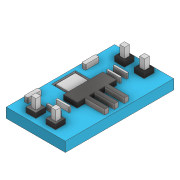
# Autodesk Inventor part: ghj
Saved by Autodesk Inventor 2021 (Build 250183000, 183)
## iProperties
Created: 2021-07-12
Part Number: ghj
Material: Generic
Document SubType Name: Modeling
Designer: Shaheen Khan
Density: 1 g/cm^3
Appearance: Default
Author: Shaheen Khan
Autodesk Inventor part; units mm, degrees
ref_plane "YZ Plane" through (0, 0, 0) normal (1, 0, 0) x (0, 1, 0)
ref_plane "XZ Plane" through (0, 0, 0) normal (0, 1, 0) x (-1, 0, 0)
ref_plane "XY Plane" through (0, 0, 0) normal (0, 0, 1) x (1, 0, 0)
sketch "Sketch1" plane through (0, 0, 0) normal (0, 1, 0) x (-1, 0, 0)
  line L0 (-15, 27.5) -> (15, 27.5)
  line L1 (15, 27.5) -> (15, -27.5)
  line L2 (15, -27.5) -> (-15, -27.5)
  line L3 (-15, -27.5) -> (-15, 27.5)
  line L4 (-15, 27.5) -> (15, -27.5) construction
  line L5 (15, 27.5) -> (-15, -27.5) construction
  point P0 (0, 0)
  dimension "d0" = 55
  dimension "d1" = 30
  constraints: 12 end point, 2 midpoint, 2 parallel, 1 horizontal, 1 perpendicular
  measures "d0" distance of L0.end L1.end
  measures "d1" distance of L1.end L2.end
extrude "Extrusion1" add sketch "Sketch1" along normal blind 5
sketch "Sketch2" plane through (0, 5, 0) normal (0, 1, 0) x (1, 0, 0)
  line L0 (-7.5, -25) -> (-2.5, -25)
  line L1 (-2.5, -25) -> (-2.5, -20)
  line L2 (-2.5, -20) -> (-7.5, -20)
  line L3 (-7.5, -20) -> (-7.5, -25)
  line L4 (-7.5, -25) -> (-2.5, -20) construction
  line L5 (-2.5, -25) -> (-7.5, -20) construction
  line L6 (-21.5261, -24.4969) -> (-16.5342, -20) construction
  line L7 (-15.0081, -24.7484) -> (-20, -20.2516) construction
  line L8 (-4.2253, 22.2548) -> (-1.8361, 26.5023) construction
  line L9 (-1.8361, 22.2548) -> (-4.2253, 26.5023) construction
  line L10 (-16.2912, 21.4805) -> (-13.725, 24.9537) construction
  line L11 (-13.725, 21.4805) -> (-16.2912, 24.9537) construction
  line L12 (-15, -27.5) -> (15, -27.5) projected
  line L13 (2.5, -25) -> (7.5, -25)
  line L14 (7.5, -25) -> (7.5, -20)
  line L15 (7.5, -20) -> (2.5, -20)
  line L16 (2.5, -20) -> (2.5, -25)
  line L17 (2.5, -25) -> (7.5, -20) construction
  line L18 (7.5, -25) -> (2.5, -20) construction
  point P0 (0, 0)
  point P1 (-5, -22.5)
  point P2 (-3.0307, 24.3785)
  point P3 (5, -22.5)
  dimension "d4" = 5
  dimension "d7" = 5
  dimension "d8" = 5
  dimension "d9" = 5
  dimension "d10" = 5
  dimension "d11" = 5
  dimension "d12" = 5
  dimension "d13" = 5
  constraints: 36 end point, 6 midpoint, 4 parallel, 2 horizontal, 2 perpendicular, 1 point on line
  measures "d4" distance from line of L12 point (-5, -22.5)
  measures "d7" horizontal distance of point (0, 0) point (-5, -22.5)
  measures "d8" distance of L1.end L2.end
  measures "d9" distance of L2.end L0.start
  measures "d10" horizontal distance of point (0, 0) point (5, -22.5)
  measures "d11" distance from line of L12 point (5, -22.5)
  measures "d12" distance of L13.start L13.end
  measures "d13" distance of L15.end L13.start
extrude "Extrusion2" add sketch "Sketch2" along normal blind 2.5
sketch "Sketch3" plane through (0, 5, 0) normal (0, 1, 0) x (1, 0, 0)
  line L0 (-7.5, 20) -> (-2.5, 20)
  line L1 (-2.5, 20) -> (-2.5, 25)
  line L2 (-2.5, 25) -> (-7.5, 25)
  line L3 (-7.5, 25) -> (-7.5, 20)
  line L4 (-7.5, 20) -> (-2.5, 25) construction
  line L5 (-2.5, 20) -> (-7.5, 25) construction
  line L6 (15, 27.5) -> (-15, 27.5) projected
  line L7 (7.5, 20) -> (2.5, 20)
  line L8 (2.5, 20) -> (2.5, 25)
  line L9 (2.5, 25) -> (7.5, 25)
  line L10 (7.5, 25) -> (7.5, 20)
  line L11 (7.5, 20) -> (2.5, 25) construction
  line L12 (2.5, 20) -> (7.5, 25) construction
  point P0 (0, 0)
  point P1 (-5, 22.5)
  point P2 (5, 22.5)
  dimension "d16" = 5
  dimension "d17" = 5
  dimension "d18" = 5
  dimension "d19" = 5
  dimension "d20" = 5
  dimension "d21" = 5
  dimension "d22" = 5
  dimension "d23" = 5
  constraints: 24 end point, 4 midpoint, 4 parallel, 2 horizontal, 2 perpendicular
  measures "d16" distance from line of L6 point (-5, 22.5)
  measures "d17" distance of L2.end L0.start
  measures "d18" distance of L0.start L0.end
  measures "d19" horizontal distance of point (0, 0) point (-5, 22.5)
  measures "d20" horizontal distance of point (0, 0) point (5, 22.5)
  measures "d21" distance of L7.start L7.end
  measures "d22" distance of L7.end L8.end
  measures "d23" distance from line of L6 point (5, 22.5)
extrude "Extrusion3" add sketch "Sketch3" along normal blind 2.5
sketch "Sketch5" plane through (0, 7.5, 0) normal (0, 1, 0) x (1, 0, 0)
  line L0 (-3.685, -23.75) -> (-6.185, -23.75)
  line L1 (-6.185, -23.75) -> (-6.185, -21.25)
  line L2 (-6.185, -21.25) -> (-3.685, -21.25)
  line L3 (-3.685, -21.25) -> (-3.685, -23.75)
  line L4 (-3.685, -23.75) -> (-6.185, -21.25) construction
  line L5 (-6.185, -23.75) -> (-3.685, -21.25) construction
  line L6 (6.452, -23.75) -> (3.952, -23.75)
  line L7 (3.952, -23.75) -> (3.952, -21.25)
  line L8 (3.952, -21.25) -> (6.452, -21.25)
  line L9 (6.452, -21.25) -> (6.452, -23.75)
  line L10 (6.452, -23.75) -> (3.952, -21.25) construction
  line L11 (3.952, -23.75) -> (6.452, -21.25) construction
  line L12 (-3.685, 21.25) -> (-6.185, 21.25)
  line L13 (-6.185, 21.25) -> (-6.185, 23.75)
  line L14 (-6.185, 23.75) -> (-3.685, 23.75)
  line L15 (-3.685, 23.75) -> (-3.685, 21.25)
  line L16 (-3.685, 21.25) -> (-6.185, 23.75) construction
  line L17 (-6.185, 21.25) -> (-3.685, 23.75) construction
  line L18 (6.452, 21.25) -> (3.952, 21.25)
  line L19 (3.952, 21.25) -> (3.952, 23.75)
  line L20 (3.952, 23.75) -> (6.452, 23.75)
  line L21 (6.452, 23.75) -> (6.452, 21.25)
  line L22 (6.452, 21.25) -> (3.952, 23.75) construction
  line L23 (3.952, 21.25) -> (6.452, 23.75) construction
  line L24 (-7.5, -25) -> (-2.5, -25) projected
  line L25 (2.5, -25) -> (7.5, -25) projected
  line L26 (-7.5, 20) -> (-2.5, 20) projected
  line L27 (2.5, 20) -> (7.5, 20) projected
  point P0 (0, 0)
  point P1 (-4.935, -22.5)
  point P2 (5.202, -22.5)
  point P3 (-4.935, 22.5)
  point P4 (5.202, 22.5)
  dimension "d34" = 2.5
  dimension "d35" = 2.5
  dimension "d36" = 2.5
  dimension "d37" = 2.5
  dimension "d38" = 2.5
  dimension "d39" = 2.5
  dimension "d40" = 2.5
  dimension "d41" = 2.5
  constraints: 48 end point, 8 midpoint, 8 parallel, 8 perpendicular, 4 horizontal, 4 point on line
  measures "d34" distance of L1.end L2.end
  measures "d35" distance of L7.end L8.end
  measures "d36" distance of L13.end L14.end
  measures "d37" distance of L19.end L20.end
  measures "d38" distance from line of L24 point (-4.935, -22.5)
  measures "d39" distance from line of L25 point (5.202, -22.5)
  measures "d40" distance from line of L26 point (-4.935, 22.5)
  measures "d41" distance from line of L27 point (5.202, 22.5)
extrude "Extrusion4" add sketch "Sketch5" along normal blind 5
sketch "Sketch6" plane through (0, 5, 0) normal (0, 1, 0) x (1, 0, 0)
  line L0 (3.5, -10) -> (-3.5, -10)
  line L1 (-3.5, -10) -> (-3.5, 10)
  line L2 (-3.5, 10) -> (3.5, 10)
  line L3 (3.5, 10) -> (3.5, -10)
  line L4 (3.5, -10) -> (-3.5, 10) construction
  line L5 (-3.5, -10) -> (3.5, 10) construction
  point P0 (0, 0)
  dimension "d44" = 20
  dimension "d45" = 7
  constraints: 12 end point, 2 midpoint, 2 parallel, 1 horizontal, 1 perpendicular
  measures "d44" distance of L0.end L1.end
  measures "d45" distance of L1.end L2.end
extrude "Extrusion5" add sketch "Sketch6" along normal blind 2.5
sketch "Sketch7" plane through (0, 5, 0) normal (0, 1, 0) x (1, 0, 0)
  line L0 (3.5, -10) -> (3.5, 10) projected
  line L1 (13.5, -6) -> (3.5, -6)
  line L2 (3.5, -6) -> (3.5, -4)
  line L3 (3.5, -4) -> (13.5, -4)
  line L4 (13.5, -4) -> (13.5, -6)
  line L5 (13.5, -6) -> (3.5, -4) construction
  line L6 (3.5, -6) -> (13.5, -4) construction
  line L7 (13.5, -1.1452) -> (3.5, -1.1452)
  line L8 (3.5, -1.1452) -> (3.5, 0.8548)
  line L9 (3.5, 0.8548) -> (13.5, 0.8548)
  line L10 (13.5, 0.8548) -> (13.5, -1.1452)
  line L11 (13.5, -1.1452) -> (3.5, 0.8548) construction
  line L12 (3.5, -1.1452) -> (13.5, 0.8548) construction
  line L13 (13.5, 4) -> (3.5, 4)
  line L14 (3.5, 4) -> (3.5, 6)
  line L15 (3.5, 6) -> (13.5, 6)
  line L16 (13.5, 6) -> (13.5, 4)
  line L17 (13.5, 4) -> (3.5, 6) construction
  line L18 (3.5, 4) -> (13.5, 6) construction
  point P0 (0, 0)
  point P1 (8.5, -5)
  point P2 (8.5, -0.1452)
  point P3 (8.5, 5)
  point P4 (3.5, 4)
  point P5 (3.5, -1.1452)
  point P6 (3.5, -6)
  dimension "d48" = 5
  dimension "d49" = 5
  dimension "d50" = 2
  dimension "d51" = 2
  dimension "d52" = 2
  dimension "d53" = 10
  dimension "d54" = 10
  dimension "d55" = 10
  constraints: 36 end point, 6 midpoint, 6 parallel, 3 horizontal, 3 perpendicular, 3 point on line
  measures "d48" horizontal distance of L0.start point (8.5, -5)
  measures "d49" horizontal distance of L0.end point (8.5, 5)
  measures "d50" distance of L3.end L1.start
  measures "d51" distance of L9.end L7.start
  measures "d52" distance of L15.end L13.start
  measures "d53" distance of L7.start L7.end
  measures "d54" distance of L1.start L1.end
  measures "d55" distance of L13.start L13.end
extrude "Extrusion6" add sketch "Sketch7" along normal blind 2.5
sketch "Sketch8" plane through (0, 5, 0) normal (0, 1, 0) x (1, 0, 0)
  line L0 (-2.5053, -4.9793) -> (-12.4638, -4.9793)
  line L1 (-12.4638, -4.9793) -> (-12.4638, 4.9793)
  line L2 (-12.4638, 4.9793) -> (-2.5053, 4.9793)
  line L3 (-2.5053, 4.9793) -> (-2.5053, -4.9793)
  line L4 (-2.5053, -4.9793) -> (-12.4638, 4.9793) construction
  line L5 (-12.4638, -4.9793) -> (-2.5053, 4.9793) construction
  line L6 (-12.4638, -4.9793) -> (-2.5053, -4.9793)
  line L7 (-2.5053, -4.9793) -> (-2.5053, 4.9793)
  line L8 (-2.5053, 4.9793) -> (-12.4638, 4.9793)
  line L9 (-12.4638, 4.9793) -> (-12.4638, -4.9793)
  line L10 (-12.4638, -4.9793) -> (-2.5053, 4.9793) construction
  line L11 (-2.5053, -4.9793) -> (-12.4638, 4.9793) construction
  line L12 (-2.779, -5.9793) -> (-13.4638, -5.9793)
  line L13 (-13.4638, -5.9793) -> (-13.4638, 5.9793)
  line L14 (-13.4638, 5.9793) -> (-2.779, 5.9793)
  line L15 (-2.779, 5.9793) -> (-2.779, -5.9793)
  line L16 (-2.779, -5.9793) -> (-13.4638, 5.9793) construction
  line L17 (-13.4638, -5.9793) -> (-2.779, 5.9793) construction
  point P0 (0, 0)
  point P1 (-7.4846, 0)
  point P2 (-8.1214, 0)
  point P3 (-2.779, -4.9793)
  point P4 (-2.779, 4.9793)
  dimension "d58" = 0
  dimension "d59" = 1
  dimension "d60" = 1
  dimension "d61" = 1
  constraints: 36 end point, 6 midpoint, 6 parallel, 3 horizontal, 3 perpendicular, 2 point on line
  measures "d58" distance between parallel lines of L3 L7
  measures "d59" distance between parallel lines of L1 L13
  measures "d60" distance between parallel lines of L12 L0
  measures "d61" distance between parallel lines of L14 L2
extrude "Extrusion7" cut sketch "Sketch8" against normal blind 1.5 contours L15 L12 L13 L14 L2 L1 L0
sketch "Sketch9" plane through (0, 5, 0) normal (0, 1, 0) x (1, 0, 0)
  line L0 (-12.9816, -20.5693) -> (-11.0184, -20.5693)
  line L1 (-11.0184, -20.5693) -> (-11.0184, -13.5693)
  line L2 (-11.0184, -13.5693) -> (-12.9816, -13.5693)
  line L3 (-12.9816, -13.5693) -> (-12.9816, -20.5693)
  line L4 (-12.9816, -20.5693) -> (-11.0184, -13.5693) construction
  line L5 (-11.0184, -20.5693) -> (-12.9816, -13.5693) construction
  line L6 (-12.9816, 8.7588) -> (-11.0184, 8.7588)
  line L7 (-11.0184, 8.7588) -> (-11.0184, 15.7588)
  line L8 (-11.0184, 15.7588) -> (-12.9816, 15.7588)
  line L9 (-12.9816, 15.7588) -> (-12.9816, 8.7588)
  line L10 (-12.9816, 8.7588) -> (-11.0184, 15.7588) construction
  line L11 (-11.0184, 8.7588) -> (-12.9816, 15.7588) construction
  line L12 (-3.4567, -19.0951) -> (-3.4567, -18.2038)
  line L13 (3.5065, -17.7666) -> (3.5065, -17.6947)
  line L14 (3.5433, -14.0693) -> (-3.4567, -14.0693)
  line L15 (-3.4567, -14.0693) -> (-3.4567, -13.0693)
  line L16 (-3.4567, -13.0693) -> (3.5433, -13.0693)
  line L17 (3.5433, -13.0693) -> (3.5433, -14.0693)
  line L18 (3.5433, -14.0693) -> (-3.4567, -13.0693) construction
  line L19 (-3.4567, -14.0693) -> (3.5433, -13.0693) construction
  line L20 (3.5433, 11.6934) -> (-3.4567, 11.6934)
  line L21 (-3.4567, 11.6934) -> (-3.4567, 12.6934)
  line L22 (-3.4567, 12.6934) -> (3.5433, 12.6934)
  line L23 (3.5433, 12.6934) -> (3.5433, 11.6934)
  line L24 (3.5433, 11.6934) -> (-3.4567, 12.6934) construction
  line L25 (-3.4567, 11.6934) -> (3.5433, 12.6934) construction
  line L26 (3.3199, 15.2588) -> (-3.6801, 15.2588)
  line L27 (-3.6801, 15.2588) -> (-3.6801, 16.2588)
  line L28 (-3.6801, 16.2588) -> (3.3199, 16.2588)
  line L29 (3.3199, 16.2588) -> (3.3199, 15.2588)
  line L30 (3.3199, 15.2588) -> (-3.6801, 16.2588) construction
  line L31 (-3.6801, 15.2588) -> (3.3199, 16.2588) construction
  line L32 (3.283, -18.5633) -> (-3.717, -18.5633)
  line L33 (-3.717, -18.5633) -> (-3.717, -17.5633)
  line L34 (-3.717, -17.5633) -> (3.283, -17.5633)
  line L35 (3.283, -17.5633) -> (3.283, -18.5633)
  line L36 (3.283, -18.5633) -> (-3.717, -17.5633) construction
  line L37 (-3.717, -18.5633) -> (3.283, -17.5633) construction
  point P0 (0, 0)
  point P1 (-12, -17.0693)
  point P2 (-12, 12.2588)
  point P3 (0.0433, -13.5693)
  point P4 (0.0433, 12.1934)
  point P5 (-0.1801, 15.7588)
  point P6 (-0.217, -18.0633)
  dimension "d64" = 1.9632
  dimension "d65" = 7
  dimension "d66" = 1.9632
  dimension "d67" = 7
  dimension "d69" = 7
  dimension "d70" = 7
  dimension "d71" = 7
  dimension "d72" = 7
  dimension "d73" = 1
  dimension "d74" = 1
  dimension "d75" = 1
  dimension "d76" = 1
  dimension "d77" = 17.0694
  dimension "d78" = 12
  dimension "d79" = 12
  dimension "d80" = 12.2588
  constraints: 76 end point, 13 parallel, 12 midpoint, 6 horizontal, 6 perpendicular, 6 point on line
  measures "d64" distance of L1.end L2.end
  measures "d65" distance of L2.end L0.start
  measures "d66" distance of L6.start L6.end
  measures "d67" distance of L8.end L6.start
  measures "d69" distance of L14.start L14.end
  measures "d70" distance of L20.start L20.end
  measures "d71" distance of L26.start L26.end
  measures "d72" distance of L32.start L32.end
  measures "d73" distance of L34.end L32.start
  measures "d74" distance of L16.end L14.start
  measures "d75" distance of L28.end L26.start
  measures "d76" distance of L22.end L20.start
  measures "d77" vertical distance of point (0, 0) point (-12, -17.069)
  measures "d78" horizontal distance of point (0, 0) point (-12, -17.069)
  measures "d79" horizontal distance of point (0, 0) point (-12, 12.259)
  measures "d80" vertical distance of point (0, 0) point (-12, 12.259)
extrude "Extrusion8" add sketch "Sketch9" along normal blind 2.5
fillet "Fillet1" radius 0.275 24 edges at (-12.9816, 6.25, 20.5693) (-11.0184, 6.25, 20.5693) (-12.9816, 6.25, 13.5693) (-11.0184, 6.25, 13.5693) (-3.717, 6.25, 18.5633) (-3.717, 6.25, 17.5633) (3.283, 6.25, 18.5633) (3.283, 6.25, 17.5633) (-3.4567, 6.25, 13.0693) (-3.4567, 6.25, 14.0693) (3.5433, 6.25, 14.0693) (3.5433, 6.25, 13.0693) (3.3199, 6.25, -15.2588) (3.3199, 6.25, -16.2588) (3.5433, 6.25, -11.6934) (3.5433, 6.25, -12.6934) (-3.4567, 6.25, -11.6934) (-3.4567, 6.25, -12.6934) (-3.6801, 6.25, -15.2588) (-3.6801, 6.25, -16.2588) (-11.0184, 6.25, -8.7588) (-12.9816, 6.25, -8.7588) (-12.9816, 6.25, -15.7588) (-11.0184, 6.25, -15.7588)
body "Solid1"
